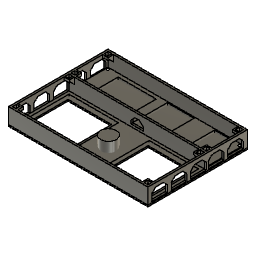
aquarium_led_cob_milieu (Autodesk Fusion 360 design; units mm, degrees)
Autodesk Fusion 360 part; units mm, degrees
sketch "Esquisse3" plane through (0, 0, 0) normal (0, 0, 1) x (1, 0, 0)
  line L0 (270, -101.5) -> (270, -108.5)
  line L1 (270, -108.5) -> (203, -108.5)
  line L2 (-7, 7) -> (270, 7)
  line L3 (270, 7) -> (270, -108.5)
  line L4 (270, -108.5) -> (-7, -108.5)
  line L5 (-7, -108.5) -> (-7, 7)
  line L6 (274, -108.5) -> (274, -112.5)
  line L7 (274, -112.5) -> (270, -112.5)
  line L8 (-11, 7) -> (-11, 11)
  line L9 (-11, 11) -> (-7, 11)
  line L10 (-11, 11) -> (274, 11)
  line L11 (274, 11) -> (274, -112.5)
  line L12 (274, -112.5) -> (-11, -112.5)
  line L13 (-11, -112.5) -> (-11, 11)
  line L14 (-11, 11) -> (274, 11)
  line L15 (274, 11) -> (274, 91)
  line L16 (274, 91) -> (-11, 91)
  line L17 (-11, 91) -> (-11, 11)
  line L18 (-11, 91) -> (-7, 91)
  line L19 (-11, 77) -> (-11, 91)
  line L20 (274, 91) -> (210, 91)
  line L21 (274, 77) -> (274, 91)
  line L22 (-7, 11) -> (-11, 11)
  line L23 (-11, 11) -> (-11, 77)
  line L24 (210, 91) -> (-7, 91)
  line L25 (274, 77) -> (274, 11)
  line L26 (-11, 91) -> (-7, 91)
  line L27 (274, 11) -> (210, 11)
  line L28 (210, 11) -> (210, 15)
  line L29 (274, 15) -> (274, 11)
  line L30 (210, 11) -> (-7, 11)
  line L31 (-7, 11) -> (-7, 87)
  line L32 (-7, 87) -> (210, 87)
  line L33 (210, 87) -> (210, 11)
  line L34 (171.3564, 84.7658) -> (116.3564, 84.7658)
  line L35 (116.3564, 84.7658) -> (116.3564, 13.7658)
  line L36 (116.3564, 13.7658) -> (171.3564, 13.7658)
  line L37 (171.3564, 13.7658) -> (171.3564, 84.7658)
  line L38 (251.3244, 84.7123) -> (213.3244, 84.7123)
  line L39 (213.3244, 84.7123) -> (213.3244, 12.7123)
  line L40 (213.3244, 12.7123) -> (251.3244, 12.7123)
  line L41 (251.3244, 12.7123) -> (251.3244, 84.7123)
  line L42 (20.6508, 79.9111) -> (98.6508, 79.9111)
  line L43 (98.6508, 79.9111) -> (98.6508, 21.9111)
  line L44 (98.6508, 21.9111) -> (20.6508, 21.9111)
  line L45 (20.6508, 21.9111) -> (20.6508, 79.9111)
  line L46 (-7, 87) -> (1, 87)
  line L47 (1, 87) -> (1, 79)
  line L48 (1, 79) -> (-7, 79)
  line L49 (-7, 79) -> (-7, 87)
  line L50 (-7, 87) -> (4, 87)
  line L51 (4, 87) -> (4, 76)
  line L52 (4, 76) -> (-7, 76)
  line L53 (-7, 76) -> (-7, 87)
  line L54 (210, 87) -> (202, 87)
  line L55 (210, 79) -> (210, 87)
  line L56 (210, 87) -> (199, 87)
  line L57 (210, 76) -> (210, 87)
  line L58 (-7, -108.5) -> (0, -108.5)
  line L59 (0, -108.5) -> (0, -100.5)
  line L60 (0, -100.5) -> (-7, -100.5)
  line L61 (-7, -100.5) -> (-7, -108.5)
  line L62 (270, -108.5) -> (262, -108.5)
  line L63 (262, -108.5) -> (262, -100.5)
  line L64 (262, -100.5) -> (270, -100.5)
  line L65 (270, -100.5) -> (270, -108.5)
  line L66 (270, -108.5) -> (259, -108.5)
  line L67 (259, -108.5) -> (259, -97.5)
  line L68 (259, -97.5) -> (270, -97.5)
  line L69 (270, -97.5) -> (270, -108.5)
  line L70 (-7, -108.5) -> (4, -108.5)
  line L71 (4, -108.5) -> (4, -97.5)
  line L72 (4, -97.5) -> (-7, -97.5)
  line L73 (-7, -97.5) -> (-7, -108.5)
  line L74 (-7, 7) -> (1, 7)
  line L75 (1, 7) -> (1, -1)
  line L76 (1, -1) -> (-7, -1)
  line L77 (-7, -1) -> (-7, 7)
  line L78 (-7, 7) -> (4, 7)
  line L79 (4, 7) -> (4, -3)
  line L80 (4, -3) -> (-7, -3)
  line L81 (-7, -3) -> (-7, 7)
  line L82 (-7, 11) -> (1, 11)
  line L83 (1, 11) -> (1, 19)
  line L84 (1, 19) -> (-7, 19)
  line L85 (-7, 11) -> (4, 11)
  line L86 (4, 11) -> (4, 22)
  line L87 (4, 22) -> (-7, 22)
  line L88 (270, 7) -> (202, 7)
  line L89 (270, -1) -> (270, 7)
  line L90 (270, 7) -> (199, 7)
  line L91 (210, 11) -> (202, 11)
  line L92 (210, 19) -> (210, 11)
  line L93 (210, 11) -> (199, 11)
  line L94 (210, 87) -> (270, 87)
  line L95 (270, 87) -> (270.0157, 11)
  line L96 (270, 87) -> (262, 87)
  line L97 (262, 87) -> (262, 79)
  line L98 (262, 79) -> (270, 79)
  line L99 (270, 79) -> (270, 87)
  line L100 (270, 87) -> (259, 87)
  line L101 (259, 87) -> (259, 76)
  line L102 (259, 76) -> (270, 76)
  line L103 (270, 76) -> (270, 87)
  line L104 (270.0157, 11) -> (262.0157, 11)
  line L105 (262.0157, 11) -> (262.0157, 19)
  line L106 (262.0157, 19) -> (270.0157, 19)
  line L107 (270.0157, 19) -> (270.0157, 11)
  line L108 (270.0157, 11) -> (259.0157, 11)
  line L109 (259.0157, 11) -> (259.0157, 22)
  line L110 (259.0157, 22) -> (270.0157, 22)
  line L111 (270, 7) -> (262, 7)
  line L112 (262, 7) -> (262, -1)
  line L113 (262, -1) -> (270, -1)
  line L114 (270, -1) -> (270, 7)
  line L115 (270, 7) -> (259, 7)
  line L116 (259, 7) -> (259, -4)
  line L117 (259, -4) -> (270, -4)
  line L118 (270, -4) -> (270, 7)
  line L119 (93, -101.5) -> (85, -101.5)
  line L120 (93, -100.5) -> (93, -101.5)
  line L121 (-7, 7) -> (-1, 7)
  line L122 (-1, 7) -> (-1, 1)
  line L123 (-1, 1) -> (-7, 1)
  line L124 (-7, 1) -> (-7, 7)
  line L125 (270, -108.5) -> (264, -108.5)
  line L126 (264, -108.5) -> (264, -102.5)
  line L127 (264, -102.5) -> (270, -102.5)
  line L128 (270, -102.5) -> (270, -108.5)
  line L129 (264, -102.5) -> (-1, -102.5)
  line L130 (-1, -102.5) -> (-1, 1)
  line L131 (-1, 1) -> (264, 1)
  line L132 (264, 1) -> (264, -102.5)
  line L133 (264, -102.5) -> (258, -102.5)
  line L134 (258, -102.5) -> (258, -96.5)
  line L135 (258, -96.5) -> (264, -96.5)
  line L136 (264, -96.5) -> (264, -102.5)
  line L137 (264, -102.5) -> (163, -102.5)
  line L138 (163, -102.5) -> (163, -1)
  line L139 (163, -1) -> (264, -1)
  line L140 (264, -1) -> (264, -102.5)
  line L141 (163, -1) -> (169, -1)
  line L142 (169, -1) -> (169, -7)
  line L143 (169, -7) -> (163, -7)
  line L144 (163, -7) -> (163, -1)
  line L145 (169, -7) -> (258, -7)
  line L146 (258, -7) -> (258, -96.5)
  line L147 (258, -96.5) -> (169, -96.5)
  line L148 (169, -96.5) -> (169, -7)
  line L149 (-1, -102.5) -> (100, -102.5)
  line L150 (100, -102.5) -> (100, -1)
  line L151 (100, -1) -> (-1, -1)
  line L152 (-1, -1) -> (-1, -102.5)
  line L153 (-1, -102.5) -> (5, -102.5)
  line L154 (5, -102.5) -> (5, -96.5)
  line L155 (5, -96.5) -> (-1, -96.5)
  line L156 (-1, -96.5) -> (-1, -102.5)
  line L157 (100, -1) -> (94, -1)
  line L158 (94, -1) -> (94, -7)
  line L159 (94, -7) -> (100, -7)
  line L160 (100, -7) -> (100, -1)
  line L161 (94, -7) -> (5, -7)
  line L162 (5, -7) -> (5, -96.5)
  line L163 (5, -96.5) -> (94, -96.5)
  line L164 (94, -96.5) -> (94, -7)
  line L165 (100, -1) -> (100, 1)
  line L166 (163, -1) -> (163, 1)
  circle A0 centre (131.5, -50.75) radius 16
  dimension "d44" = 4
  dimension "d45" = 4
  dimension "d46" = 4
  dimension "d47" = 4
  dimension "d48" = 285
  dimension "d49" = 80
  dimension "d62" = 55
  dimension "d63" = 71
  dimension "d64" = 38
  dimension "d65" = 72
  dimension "d66" = 78
  dimension "d67" = 58
  dimension "d92" = 8
  dimension "d93" = 8
  dimension "d94" = 11
  dimension "d95" = 11
  dimension "d96" = 8
  dimension "d98" = 11
  dimension "d100" = 7
  dimension "d101" = 8
  dimension "d102" = 8
  dimension "d103" = 8
  dimension "d104" = 11
  dimension "d105" = 11
  dimension "d106" = 11
  dimension "d155" = 217
  dimension "d156" = 285
  dimension "d157" = 11
  dimension "d159" = 8
  dimension "d160" = 8
  dimension "d161" = 11
  dimension "d162" = 11
  dimension "d164" = 8
  dimension "d166" = 11
  dimension "d167" = 8
  dimension "d168" = 8
  dimension "d169" = 11
  dimension "d170" = 11
  dimension "d180" = 6
  dimension "d181" = 6
  dimension "d182" = 6
  dimension "d183" = 6
  dimension "d184" = 101
  dimension "d185" = 101.5
  dimension "d186" = 6
  dimension "d187" = 6
  dimension "d188" = 101
  dimension "d189" = 101.5
  dimension "d190" = 6
  dimension "d191" = 6
  dimension "d192" = 6
  dimension "d193" = 6
  dimension "d247" = 32
  constraint vertical L0
  constraint horizontal L1
  constraint horizontal L2
  constraint vertical L3
  constraint horizontal L4
  constraint vertical L5
  constraint vertical L6
  constraint horizontal L7
  constraint vertical L8
  constraint horizontal L9
  constraint horizontal L10
  constraint vertical L11
  constraint horizontal L12
  constraint vertical L13
  constraint horizontal L14
  constraint vertical L15
  constraint horizontal L16
  constraint vertical L17
  constraint horizontal L18
  constraint vertical L19
  constraint horizontal L20
  constraint vertical L21
  constraint horizontal L22
  constraint vertical L23
  constraint horizontal L24
  constraint vertical L25
  constraint horizontal L26
  constraint horizontal L27
  constraint vertical L28
  constraint vertical L29
  constraint horizontal L30
  constraint vertical L31
  constraint horizontal L32
  constraint vertical L33
  constraint horizontal L34
  constraint vertical L35
  constraint horizontal L36
  constraint vertical L37
  constraint horizontal L38
  constraint vertical L39
  constraint horizontal L40
  constraint vertical L41
  constraint horizontal L42
  constraint vertical L43
  constraint horizontal L44
  constraint vertical L45
  constraint horizontal L46
  constraint vertical L47
  constraint horizontal L48
  constraint vertical L49
  constraint horizontal L50
  constraint vertical L51
  constraint horizontal L52
  constraint vertical L53
  constraint horizontal L54
  constraint vertical L55
  constraint horizontal L56
  constraint vertical L57
  constraint horizontal L58
  constraint vertical L59
  constraint horizontal L60
  constraint vertical L61
  constraint horizontal L62
  constraint vertical L63
  constraint horizontal L64
  constraint vertical L65
  constraint horizontal L66
  constraint vertical L67
  constraint horizontal L68
  constraint vertical L69
  constraint horizontal L70
  constraint vertical L71
  constraint horizontal L72
  constraint vertical L73
  constraint horizontal L74
  constraint vertical L75
  constraint horizontal L76
  constraint vertical L77
  constraint horizontal L78
  constraint vertical L79
  constraint horizontal L80
  constraint vertical L81
  constraint horizontal L82
  constraint vertical L83
  constraint horizontal L84
  constraint horizontal L85
  constraint vertical L86
  constraint horizontal L87
  constraint horizontal L88
  constraint vertical L89
  constraint horizontal L90
  constraint horizontal L91
  constraint vertical L92
  constraint horizontal L93
  constraint perpendicular L57 L94
  constraint coincident L14 L95.end
  constraint horizontal L96
  constraint vertical L97
  constraint horizontal L98
  constraint vertical L99
  constraint horizontal L100
  constraint vertical L101
  constraint horizontal L102
  constraint vertical L103
  constraint horizontal L104
  constraint vertical L105
  constraint horizontal L106
  constraint vertical L107
  constraint horizontal L108
  constraint vertical L109
  constraint horizontal L110
  constraint horizontal L111
  constraint vertical L112
  constraint horizontal L113
  constraint vertical L114
  constraint horizontal L115
  constraint vertical L116
  constraint horizontal L117
  constraint vertical L118
  constraint horizontal L119
  constraint vertical L120
  constraint horizontal L121
  constraint vertical L122
  constraint horizontal L123
  constraint vertical L124
  constraint horizontal L125
  constraint vertical L126
  constraint horizontal L127
  constraint vertical L128
  constraint horizontal L129
  constraint vertical L130
  constraint horizontal L131
  constraint vertical L132
  constraint horizontal L133
  constraint vertical L134
  constraint horizontal L135
  constraint vertical L136
  constraint horizontal L137
  constraint vertical L138
  constraint horizontal L139
  constraint vertical L140
  constraint horizontal L141
  constraint vertical L142
  constraint horizontal L143
  constraint vertical L144
  constraint horizontal L145
  constraint vertical L146
  constraint horizontal L147
  constraint vertical L148
  constraint horizontal L149
  constraint vertical L150
  constraint horizontal L151
  constraint vertical L152
  constraint horizontal L153
  constraint vertical L154
  constraint horizontal L155
  constraint vertical L156
  constraint horizontal L157
  constraint vertical L158
  constraint horizontal L159
  constraint vertical L160
  constraint horizontal L161
  constraint vertical L162
  constraint horizontal L163
  constraint vertical L164
  constraint coincident L131 L165.end
  constraint perpendicular L131 L165
  constraint coincident L131 L166.end
  constraint perpendicular L131 L166
  measures "d44" distance of L0.end L6.start
  measures "d45" distance of L0.end L7.end
  measures "d46" distance of L2.start L8.start
  measures "d47" distance of L2.start L9.end
  measures "d48" distance of L8.end L10.end
  measures "d49" distance of L8.end L16.end
  measures "d62" distance of L34.start L34.end
  measures "d63" distance of L34.start L36.end
  measures "d64" distance of L38.start L38.end
  measures "d65" distance of L38.start L40.end
  measures "d66" distance of L42.start L42.end
  measures "d67" distance of L42.start L44.end
  measures "d92" distance of L31.end L46.end
  measures "d93" distance of L31.end L48.end
  measures "d94" distance of L31.end L50.end
  measures "d95" distance of L31.end L52.end
  measures "d96" distance of L32.end L54.end
  measures "d98" distance of L32.end L56.end
  measures "d100" distance of L4.end L58.end
  measures "d101" distance of L4.end L60.end
  measures "d102" distance of L0.end L62.end
  measures "d103" distance of L0.end L64.end
  measures "d104" distance of L0.end L66.end
  measures "d105" distance of L4.end L70.end
  measures "d106" distance of L4.end L72.end
  measures "d155" distance of L27.end L9.end
  measures "d156" distance of L8.end L10.end
  measures "d157" distance of L67.end L68.end
  measures "d159" distance of L94.end L96.end
  measures "d160" distance of L94.end L98.end
  measures "d161" distance of L94.end L100.end
  measures "d162" distance of L94.end L102.end
  measures "d164" distance of L95.end L106.end
  measures "d166" distance of L95.end L110.end
  measures "d167" distance of L2.end L111.end
  measures "d168" distance of L2.end L89.start
  measures "d169" distance of L2.end L115.end
  measures "d170" distance of L2.end L117.end
  measures "d180" distance of L0.end L125.end
  measures "d181" distance of L0.end L127.end
  measures "d182" distance of L126.end L133.end
  measures "d183" distance of L126.end L135.end
  measures "d184" distance of L126.end L137.end
  measures "d185" distance of L126.end L139.end
  measures "d186" distance of L138.end L141.end
  measures "d187" distance of L138.end L143.end
  measures "d188" distance of L129.end L149.end
  measures "d189" distance of L129.end L151.end
  measures "d190" distance of L129.end L153.end
  measures "d191" distance of L129.end L155.end
  measures "d192" distance of L150.end L157.end
  measures "d193" distance of L150.end L159.end
  measures "d247" diameter of A0
extrude "Extrusion19" add sketch "Esquisse3" along normal blind 25 contours A0 makes body 1
sketch "Esquisse6" plane through (0, 7, 0) normal (0, -1, 0) x (1, 0, 0)
  line L0 (-7, 19.25) -> (-11, 19.25)
  line L1 (-11, 19.25) -> (-11, 5.25)
  line L2 (-11, 5.25) -> (-7, 5.25)
  line L3 (-7, 5.25) -> (-7, 0)
  line L4 (-7, 0) -> (270, 0)
  line L5 (270, 0) -> (270, 35)
  line L6 (270, 35) -> (259, 35)
  line L7 (-7, 35) -> (-7, 19.25)
  line L8 (90, 30) -> (110, 30)
  line L9 (110, 30) -> (110, 20)
  line L10 (110, 20) -> (90, 20)
  line L11 (90, 20) -> (90, 30)
  line L12 (259, 30) -> (1, 30)
  line L13 (1, 30) -> (1, 35)
  line L14 (1, 35) -> (-7, 35)
  line L15 (259, 35) -> (259, 30)
  constraint horizontal L8
  constraint vertical L9
  constraint horizontal L10
  constraint vertical L11
extrude "Extrusion12" add sketch "Esquisse3" along normal blind 5.25 separate body contours L0 L3 L64 L65 L69 L127 L132 L136 L140 | L0 L1 L3 L4 L62 L65 L66 L69 L125 L126 L127 L128 | L3 L64 L68 L69 L132 L136 L140 | L1 L4 L62 L63 L66 L126 L129 L133 L137 | L3 L68 L117 L132 L136 L140 | L1 L4 L63 L66 L67 L129 L133 L137 | L3 L113 L117 L118 L132 L140 | L1 L4 L67 L71 L129 L133 L137 L149 L153 | L2 L3 L88 L89 L90 L111 L112 L113 L114 L115 L118 L131 L132 | L129 L131 L138 L144 L150 L160 L165 L166 | L2 L88 L90 L112 L115 L116 L131 | L4 L59 L70 L71 L129 L149 L153 | L2 L79 L88 L90 L116 L131 | L4 L5 L58 L59 L60 L61 L70 L73 L129 L130 L149 L152 L153 L156 | L5 L60 L72 L73 L130 L152 L156 | L5 L72 L80 L130 L152 L156 | L2 L75 L78 L79 L131 | L5 L76 L80 L81 L130 L152 | L2 L74 L75 L78 L122 L131 | L5 L76 L77 L81 L123 L130 | L2 L5 L74 L77 L78 L81 L121 L122 L123 L124 | A0 makes body 2
extrude "Extrusion13" add sketch "Esquisse3" along normal blind 7 separate body contours L10 L14 L27 L95 L104 L105 L106 L107 L108 | L10 L14 L27 L95 L105 L106 L108 L109 L110 | L10 L14 L27 L28 L33 L55 L57 L92 L94 L95 L101 L102 L103 L109 L110 | L10 L14 L28 L30 L31 L32 L33 L51 L52 L54 L55 L56 L57 L86 L87 L91 L92 L93 | L94 L95 L96 L97 L98 L99 L100 L103 | L94 L97 L98 L100 L101 L102 L103 | L10 L14 L30 L31 L82 L83 L84 L85 | L10 L14 L30 L31 L83 L84 L85 L86 L87 | L31 L32 L47 L48 L50 L51 L52 L53 | L31 L32 L46 L47 L48 L49 L50 L53 makes body 3
extrude "Extrusion14" add sketch "Esquisse3" along normal blind 35 separate body contours L6 L7 L8 L9 L10 L11 L12 L13 L14 L22 L27 L30 L82 L85 L91 L93 L104 L108 | L9 L10 L14 L15 L16 L17 L18 L19 L20 L21 L22 L23 L24 L25 L26 L27 L29 L31 L32 L46 L49 L50 L53 L54 L56 L94 L95 L96 L99 L100 L103 L107 makes body 4
sketch "Esquisse7" plane through (-11, 0, 0) normal (-1, 0, 0) x (0, -1, 0)
  line L0 (-91, 0) -> (112.5, 0)
  line L1 (112.5, 0) -> (112.5, 35)
  line L2 (112.5, 35) -> (-91, 35)
  line L3 (-91, 35) -> (-91, 0)
  line L4 (-91, 0) -> (112.5, 0)
  line L5 (112.5, 0) -> (112.5, 5.25)
  line L6 (112.5, 5.25) -> (-91, 5.25)
  line L7 (-91, 5.25) -> (-91, 0)
  line L8 (112.5, 5.25) -> (104.5, 5.25)
  line L9 (104.5, 5.25) -> (104.5, 27.25)
  line L10 (104.5, 27.25) -> (112.5, 27.25)
  line L11 (112.5, 27.25) -> (112.5, 5.25)
  line L12 (104.5, 27.25) -> (72.7, 27.25)
  line L13 (72.7, 27.25) -> (72.7, 5.25)
  line L14 (72.7, 5.25) -> (104.5, 5.25)
  line L15 (104.5, 5.25) -> (104.5, 27.25)
  line L16 (72.7, 27.25) -> (64.7, 27.25)
  line L17 (64.7, 27.25) -> (64.7, 5.25)
  line L18 (64.7, 5.25) -> (72.7, 5.25)
  line L19 (72.7, 5.25) -> (72.7, 27.25)
  line L20 (64.7, 27.25) -> (32.9, 27.25)
  line L21 (32.9, 27.25) -> (32.9, 5.25)
  line L22 (32.9, 5.25) -> (64.7, 5.25)
  line L23 (64.7, 5.25) -> (64.7, 27.25)
  line L24 (32.9, 27.25) -> (24.9, 27.25)
  line L25 (24.9, 27.25) -> (24.9, 5.25)
  line L26 (24.9, 5.25) -> (32.9, 5.25)
  line L27 (32.9, 5.25) -> (32.9, 27.25)
  line L28 (24.9, 27.25) -> (-6.9, 27.25)
  line L29 (-6.9, 27.25) -> (-6.9, 5.25)
  line L30 (-6.9, 5.25) -> (24.9, 5.25)
  line L31 (24.9, 5.25) -> (24.9, 27.25)
  line L32 (-11.1, 27.25) -> (-11.1, 5.25)
  line L33 (-11.1, 5.25) -> (-6.9, 5.25)
  line L34 (-6.9, 5.25) -> (-6.9, 27.25)
  line L35 (-11.1, 27.25) -> (-42.8, 27.25)
  line L36 (-42.8, 27.25) -> (-42.8, 5.25)
  line L37 (-42.8, 5.25) -> (-11.1, 5.25)
  line L38 (-11.1, 5.25) -> (-11.1, 27.25)
  line L39 (-42.8, 27.25) -> (-50.8, 27.25)
  line L40 (-50.8, 27.25) -> (-50.8, 5.25)
  line L41 (-50.8, 5.25) -> (-42.8, 5.25)
  line L42 (-42.8, 5.25) -> (-42.8, 27.25)
  line L43 (-50.8, 27.25) -> (-82.6, 27.25)
  line L44 (-82.6, 27.25) -> (-82.6, 5.25)
  line L45 (-82.6, 5.25) -> (-50.8, 5.25)
  line L46 (-50.8, 5.25) -> (-50.8, 27.25)
  line L47 (-82.6, 27.25) -> (-91, 27.25)
  line L48 (-91, 27.25) -> (-91, 5.25)
  line L49 (-91, 5.25) -> (-82.6, 5.25)
  line L50 (-82.6, 5.25) -> (-82.6, 27.25)
  dimension "d205" = 5.25
  dimension "d206" = 8
  dimension "d207" = 22
  dimension "d208" = 31.8
  dimension "d209" = 8
  dimension "d210" = 31.8
  dimension "d211" = 8
  dimension "d212" = 31.8
  dimension "d214" = 31.7
  dimension "d215" = 8
  dimension "d216" = 31.8
  constraint horizontal L4
  constraint vertical L5
  constraint horizontal L6
  constraint vertical L7
  constraint coincident L0.start L3.end
  constraint horizontal L8
  constraint vertical L9
  constraint horizontal L10
  constraint vertical L11
  constraint horizontal L12
  constraint vertical L13
  constraint horizontal L14
  constraint vertical L15
  constraint horizontal L16
  constraint vertical L17
  constraint horizontal L18
  constraint vertical L19
  constraint horizontal L20
  constraint vertical L21
  constraint horizontal L22
  constraint vertical L23
  constraint horizontal L24
  constraint vertical L25
  constraint horizontal L26
  constraint vertical L27
  constraint horizontal L28
  constraint vertical L29
  constraint horizontal L30
  constraint vertical L31
  constraint vertical L32
  constraint horizontal L33
  constraint vertical L34
  constraint horizontal L35
  constraint vertical L36
  constraint horizontal L37
  constraint vertical L38
  constraint horizontal L39
  constraint vertical L40
  constraint horizontal L41
  constraint vertical L42
  constraint horizontal L43
  constraint vertical L44
  constraint horizontal L45
  constraint vertical L46
  constraint horizontal L47
  constraint vertical L48
  constraint horizontal L49
  constraint vertical L50
  measures "d205" distance of L0.start L6.end
  measures "d206" distance of L5.end L8.end
  measures "d207" distance of L5.end L10.end
  measures "d208" distance of L9.end L12.end
  measures "d209" distance of L12.end L16.end
  measures "d210" distance of L16.end L20.end
  measures "d211" distance of L20.end L24.end
  measures "d212" distance of L24.end L28.end
  measures "d214" distance of L32.start L35.end
  measures "d215" distance of L35.end L39.end
  measures "d216" distance of L39.end L43.end
extrude "Extrusion17" cut sketch "Esquisse7" against normal blind 310 contours L6 L40 L43 L44 L45 L46 L50 | L6 L9 L12 L13 L14 L15 L19 | L6 L32 L35 L36 L37 L38 L42 | L6 L17 L20 L21 L22 L23 L27 | L6 L25 L28 L29 L30 L31 L34 bodies 4
extrude "Extrusion15" add sketch "Esquisse3" along normal blind 3 separate body contours L0 L3 L64 L65 L69 L127 L132 L136 L140 | L0 L1 L3 L4 L62 L65 L66 L69 L125 L126 L127 L128 | L3 L64 L68 L69 L132 L136 L140 | L1 L4 L62 L63 L66 L126 L129 L133 L137 | L63 L64 L129 L132 L133 L136 L137 L140 | L3 L68 L117 L132 L136 L140 | L63 L64 L67 L68 L129 L132 L133 L136 L137 L140 | L1 L4 L63 L66 L67 L129 L133 L137 | L3 L113 L117 L118 L132 L140 | L67 L68 L129 L132 L133 L134 L135 L136 L137 L140 | L1 L4 L67 L71 L129 L133 L137 L149 L153 | L2 L3 L88 L89 L90 L111 L112 L113 L114 L115 L118 L131 L132 | L116 L117 L132 L135 L139 L140 L142 L145 L146 | L113 L116 L117 L132 L139 L140 | L129 L134 L137 L138 L143 L147 L148 | L112 L113 L131 L132 L139 | L129 L131 L138 L144 L150 L160 L165 L166 | L2 L88 L90 L112 L115 L116 L131 | L112 L116 L131 L139 | L116 L131 L139 L141 L166 | L4 L59 L70 L71 L129 L149 L153 | L129 L149 L150 L154 L159 L163 L164 | L138 L139 L141 L142 L143 L144 | L2 L79 L88 L90 L116 L131 | L4 L5 L58 L59 L60 L61 L70 L73 L129 L130 L149 L152 L153 L156 | L59 L60 L71 L72 L129 L130 L149 L152 L153 L156 | L71 L72 L129 L130 L149 L152 L153 L154 L155 L156 | L150 L151 L157 L158 L159 L160 | L59 L60 L129 L130 L149 L152 L153 L156 | L79 L80 L130 L151 L152 L155 L158 L161 L162 | L79 L131 L151 L157 L165 | L5 L60 L72 L73 L130 L152 L156 | L5 L72 L80 L130 L152 L156 | L2 L75 L78 L79 L131 | L75 L79 L131 L151 | L76 L79 L80 L130 L151 L152 | L5 L76 L80 L81 L130 L152 | L2 L74 L75 L78 L122 L131 | L75 L76 L130 L131 L151 | L5 L76 L77 L81 L123 L130 | L2 L5 L74 L77 L78 L81 L121 L122 L123 L124 | L6 L7 L8 L9 L10 L11 L12 L13 L14 L22 L27 L30 L82 L85 L91 L93 L104 L108 | L9 L10 L14 L15 L16 L17 L18 L19 L20 L21 L22 L23 L24 L25 L26 L27 L29 L31 L32 L46 L49 L50 L53 L54 L56 L94 L95 L96 L99 L100 L103 L107 | L10 L14 L27 L28 L33 L55 L57 L92 L94 L95 L101 L102 L103 L109 L110 | L10 L14 L28 L30 L31 L32 L33 L51 L52 L54 L55 L56 L57 L86 L87 L91 L92 L93 | L94 L95 L96 L97 L98 L99 L100 L103 | L94 L97 L98 L100 L101 L102 L103 | L10 L14 L30 L31 L82 L83 L84 L85 | L10 L14 L30 L31 L83 L84 L85 L86 L87 | L31 L32 L47 L48 L50 L51 L52 L53 | L31 L32 L46 L47 L48 L49 L50 L53 | L34 L35 L36 L37 | L38 L39 L40 L41 | L42 L43 L44 L45 | A0 makes body 5
extrude "Extrusion16" add sketch "Esquisse3" along normal blind 5 from surface at 30 contours L3 L64 L68 L69 L132 L136 L140 | L63 L64 L67 L68 L129 L132 L133 L136 L137 L140 | L1 L4 L63 L66 L67 L129 L133 L137 | L3 L113 L117 L118 L132 L140 | L113 L116 L117 L132 L139 L140 | L2 L88 L90 L112 L115 L116 L131 | L112 L116 L131 L139 | L4 L59 L70 L71 L129 L149 L153 | L59 L60 L71 L72 L129 L130 L149 L152 L153 L156 | L5 L60 L72 L73 L130 L152 L156 | L2 L75 L78 L79 L131 | L75 L79 L131 L151 | L76 L79 L80 L130 L151 L152 | L5 L76 L80 L81 L130 L152 | L10 L14 L27 L95 L105 L106 L108 L109 L110 | L94 L97 L98 L100 L101 L102 L103 | L10 L14 L30 L31 L83 L84 L85 L86 L87 | L31 L32 L47 L48 L50 L51 L52 L53 bodies 4
chamfer "Chanfrein7" distance 8 angle 45 21 edges at (272.0005, 82.6, 27.25) (272.0046, 42.8, 27.25) (272, 6.9, 27.25) (272, -32.9, 27.25) (272, -72.7, 27.25) (272.0037, 50.8, 27.25) (272.0078, 11.1, 27.25) (-9, 11.1, 27.25) (272, -24.9, 27.25) (272, -64.7, 27.25) (272, -104.5, 27.25) (-9, -72.7, 27.25) (-9, -32.9, 27.25) (-9, 6.9, 27.25) (-9, 42.8, 27.25) (-9, 82.6, 27.25) (-9, 50.8, 27.25) (-9, 11.1, 27.25) (-9, -24.9, 27.25) (-9, -64.7, 27.25) (-9, -104.5, 27.25) on bodies 4
hole "Perçage10" at (71.9023, 15.5538, 7) direction (0, 0, -1) diameter 5.5 depth 40 tip angle 180 bodies 3 5
hole "Perçage14" at (80.303, 15.3984, 7) direction (0, 0, -1) diameter 5.5 depth 40 tip angle 180 bodies 3 5
hole "Perçage15" at (87.8237, 15.5619, 7) direction (0, 0, -1) diameter 5.5 depth 40 tip angle 180 bodies 3 5
hole "Perçage16" at (95.6713, 15.3984, 7) direction (0, 0, -1) diameter 5.5 depth 40 tip angle 180 bodies 3 5
sketch "Esquisse8" plane through (0, 7, 0) normal (0, -1, 0) x (1, 0, 0)
  line L0 (-7, 0) -> (270, 0)
  line L1 (270, 0) -> (270, 35)
  line L2 (1, 35) -> (-7, 35)
  line L3 (-7, 35) -> (-7, 0)
  line L4 (120, 10) -> (145, 10)
  line L5 (145, 10) -> (145, 25)
  line L6 (145, 25) -> (120, 25)
  line L7 (120, 25) -> (120, 10)
  line L8 (4, 35) -> (4, 30)
  line L9 (4, 30) -> (1, 30)
  line L10 (1, 30) -> (1, 35)
  line L11 (270, 35) -> (262, 35)
  line L12 (262, 35) -> (262, 30)
  line L13 (262, 30) -> (259, 30)
  line L14 (259, 30) -> (259, 35)
  line L15 (259, 35) -> (4, 35)
  dimension "d244" = 15
  constraint horizontal L4
  constraint vertical L5
  constraint horizontal L6
  constraint vertical L7
  measures "d244" distance of L4.end L5.end
extrude "Extrusion18" cut sketch "Esquisse8" against normal blind 12 contours L4 L5 L6 L7 bodies 4
chamfer "Chanfrein8" distance 8 angle 45 2 edges at (120, 9, 25) (145, 9, 25) on bodies 4
chamfer "Chanfrein9" distance 8 angle 45 4 edges at (260.5, 7, 30) (2.5, 7, 30) (2, -108.5, 30) (260.5, -108.5, 30) on bodies 4
chamfer "Chanfrein10" distance 2.84 angle 45 4 edges at (270, -99, 30) (270, -2.5, 30) (-7, -2, 30) (-7, -99, 30) on bodies 4
chamfer "Chanfrein11" distance 8 angle 45 4 edges at (260.5, 87, 30) (260.5157, 11, 30) (2.5, 11, 30) (2.5, 87, 30) on bodies 4
chamfer "Chanfrein12" distance 2.84 angle 45 2 edges at (-7, 77.5, 30) (-7, 20.5, 30) on bodies 4
chamfer "Chanfrein13" distance 2.84 angle 45 2 edges at (270.0137, 20.5, 30) (270, 77.5, 30) on bodies 4
hole "Perçage17" at (265.8258, 82.9315, 7) direction (0, 0, -1) diameter 5.035 depth 40 tip angle 180 bodies 3 5
thread "Filetage6" "ISO Metric profile 6.0 M6x1 6H"
hole "Perçage18" at (265.6951, -104.5529, 5.25) direction (0, 0, -1) diameter 5.035 depth 40 tip angle 180 bodies 2 5
thread "Filetage7" "ISO Metric profile 6.0 M6x1 6H"
hole "Perçage19" at (-3.2041, -104.5037, 5.25) direction (0, 0, -1) diameter 5.035 depth 40 tip angle 180 bodies 2 5
thread "Filetage8" "ISO Metric profile 6.0 M6x1 6H"
hole "Perçage20" at (-3.4, 83.1925, 7) direction (0, 0, -1) diameter 5.035 depth 40 tip angle 180 bodies 3 5
thread "Filetage9" "ISO Metric profile 6.0 M6x1 6H"
